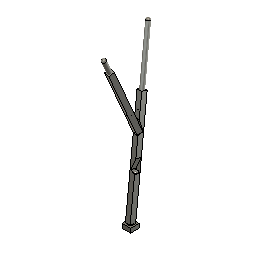
TT-4 (Autodesk Fusion 360 design; units mm, degrees)
Autodesk Fusion 360 part; units mm, degrees
sketch "Sketch1" plane through (0, 0, 0) normal (0, 1, 0) x (1, 0, 0) in component "TT-2 v5"
  line L0 (2.5, -2.5) -> (-2.5, -2.5)
  line L1 (-2.5, -2.5) -> (-2.5, 2.5)
  line L2 (-2.5, 2.5) -> (2.5, 2.5)
  line L3 (2.5, 2.5) -> (2.5, -2.5)
  constraint horizontal L0
  constraint vertical L1
  constraint horizontal L2
  constraint vertical L3
extrude "Extrude1" add sketch "Sketch1" along normal blind 2.5 makes body 1 in component "TT-2 v5"
sketch "Sketch2" plane through (0, 0, 0) normal (0, 1, 0) x (1, 0, 0) in component "TT-2 v5"
  line L0 (1.5, -1.5) -> (-1.5, -1.5)
  line L1 (-1.5, -1.5) -> (-1.5, 1.5)
  line L2 (-1.5, 1.5) -> (1.5, 1.5)
  line L3 (1.5, 1.5) -> (1.5, -1.5)
  constraint horizontal L0
  constraint vertical L1
  constraint horizontal L2
  constraint vertical L3
extrude "Extrude2" add sketch "Sketch2" along normal blind 60 separate body makes body 2 in component "TT-2 v5"
move_body "Move1" bodies 2 to x (0.939693, -0.34202, 0) y (0.34202, 0.939693, 0) z (0, 0, 1) at (-0.0905, -0.513, 0) in component "TT-2 v5"
move_body "Move2" bodies 2 to x (1, 0, 0) y (0, 1, 0) z (0, 0, 1) at (3.3727, 9.6612, 0) in component "TT-2 v5"
sphere "SpherePrimitive1" add diameter 3 placed x (0, 0, 1) y (-0.939693, 0.34202, 0) z (-0.34202, -0.939693, 0) at (3.3241, 9.1329, 0) bodies 2 in component "TT-2 v5"
sphere "SpherePrimitive2" cut diameter 3 placed x (-1, 0, 0) y (0, 0, 1) z (0, 1, 0) at (0, 2.5, 0) bodies 1 in component "TT-2 v5"
cylinder "CylinderPrimitive1" add diameter 2.5 height 40 placed x (0.883022, -0.321394, -0.34202) y (-0.321394, 0.116978, -0.939693) z (0.34202, 0.939693, 0) at (23.8453, 65.5145, 0) separate body makes body 3 in component "TT-2 v5"
sphere "SpherePrimitive3" add diameter 2.5 placed x (0, 0, -1) y (-0.939693, 0.34202, 0) z (0.34202, 0.939693, 0) at (37.5261, 103.1022, 0) bodies 3 in component "TT-2 v5"
move_body "Move3" bodies 3 2 to x (0.939693, 0.34202, 0) y (-0.34202, 0.939693, 0) z (0, 0, 1) at (23.6283, -3.8286, 0) in component "TT-2 v5"
move_body "Move4" bodies 2 3 to x (1, 0, 0) y (0, 1, 0) z (0, 0, 1) at (-23.6681, -3.196, 0) in component "TT-2 v5"
copy_body "CopyPasteBodies1" bodies 3 2 makes body 4 makes body 5 in component "TT-2 v5"
move_body "Move5" bodies 4 5 to x (1, 0, 0) y (0, 0.906308, 0.422618) z (0, -0.422618, 0.906308) at (0, 42.015, -10.6133) in component "TT-2 v5"
move_body "Move6" bodies 5 4 to x (1, 0, 0) y (0, 1, 0) z (0, 0, 1) at (0, -2.8403, 9.6134) in component "TT-2 v5"
extrude "Extrude3" cut 1 faces at (0.4157, 96.2065, 25.0427) along direction (0, -0.906308, -0.422618) blind 15 on bodies 5 bodies 5 in component "TT-2 v5"
move_body "Move7" bodies 4 to x (1, 0, 0) y (0, 1, 0) z (0, 0, 1) at (0, -26.7116, -12.4558) in component "TT-2 v5"
move_body "Move8" bodies 5 4 to x (1, 0, 0) y (0, 1, 0) z (0, 0, 1) at (0, -15.5908, 0) in component "TT-2 v5"
copy_body "CopyPasteBodies2" bodies 4 5 makes body 6 makes body 7 in component "TT-2 v5"
move_body "Move9" bodies 6 7 to x (0, 0, -1) y (0, 1, 0) z (1, 0, 0) at (-0.0791, 0, -0.06) in component "TT-2 v5"
move_body "Move10" bodies 6 to x (1, 0, 0) y (0, 1, 0) z (0, 0, 1) at (5.2397, 11.2365, 0) in component "TT-2 v5"
move_body "Move11" bodies 7 3 4 2 5 6 to x (1, 0, 0) y (0, 0.984808, -0.173648) z (0, 0.173648, 0.984808) at (0, 0.0409, 0.4679) in component "TT-2 v5"
move_body "Move12" bodies 5 4 to x (1, 0, 0) y (0, 1, 0) z (0, 0, 1) at (0, 17.3834, -3.0131) in component "TT-2 v5"
sketch "Sketch7" plane through (0, 0, 0) normal (0, 1, 0) x (1, 0, 0) in component "TT-2 v5"
  line L0 (20, -30) -> (50, 15)
  line L1 (50, 15) -> (20, 47.2574)
  line L2 (20, 47.2574) -> (-26.886, 18.4817)
  line L3 (-26.886, 18.4817) -> (-3.443, -34.2088)
  line L4 (-3.443, -34.2088) -> (20, -30)
extrude "Extrude4" add sketch "Sketch7" along normal blind 2 separate body makes body 8 in component "TT-2 v5"
move_body "Move13" bodies 8 to x (1, 0, 0) y (0, 1, 0) z (0, 0, 1) at (0, 114.7446, 0) in component "TT-2 v5"
sketch "Sketch8" plane through (0, 114.7446, 0) normal (0, -1, 0) x (1, 0, 0) in component "TT-2 v5"
  line L0 (20, 30) -> (-3.443, 34.2088)
  line L1 (-3.443, 34.2088) -> (-26.886, -18.4817)
  line L2 (-26.886, -18.4817) -> (20, -47.2574)
  line L3 (20, -47.2574) -> (50, -15)
  line L4 (50, -15) -> (20, 30)
sphere "SpherePrimitive4" cut diameter 2.5 placed x (1, 0, 0) y (0, 0, 1) z (0, -1, 0) at (-5, 114.7446, -17) bodies 8 in component "TT-2 v5"
sphere "SpherePrimitive5" cut diameter 2.5 placed x (1, 0, 0) y (0, 0, 1) z (0, -1, 0) at (3, 114.7446, 17) bodies 8 in component "TT-2 v5"
sphere "SpherePrimitive6" cut diameter 2.5 placed x (1, 0, 0) y (0, 0, 1) z (0, -1, 0) at (32.239, 114.7446, -14.3242) bodies 8 in component "TT-2 v5"
copy_body "CopyPasteBodies3" bodies 7 5 makes body 9 makes body 10 in component "TT-2 v5"
extrude "Extrude5" cut 1 faces at (19.5306, 65.7186, -10.5804) along direction (-0.422618, -0.892539, 0.157379) blind 45 on bodies 9 bodies 9 in component "TT-2 v5"
extrude "Extrude6" cut 1 faces at (-0.5843, 86.4162, 5.2019) along direction (0, -0.965926, -0.258819) blind 45 on bodies 10 bodies 10 in component "TT-2 v5"
combine "Combine1" operation cut target body 2 tool bodies 9 in component "TT-2 v5"
combine "Combine2" operation cut target body 2 tool bodies 10 in component "TT-2 v5"
copy_body "CopyPasteBodies4" bodies 7 5 makes body 11 makes body 12 in component "TT-2 v5"
combine "Combine3" operation cut target body 2 tool bodies 11 12 in component "TT-2 v5"
copy_body "Body->Comp1" bodies 1 removing the originals makes body 13 in component "MainFix"
copy_body "Body->Comp2" bodies 3 removing the originals makes body 14 in component "MainAct"
copy_body "Body->Comp3" bodies 4 removing the originals makes body 15 in component "LeftAct"
copy_body "Body->Comp4" bodies 2 removing the originals makes body 16 in component "MainBranch"
copy_body "Body->Comp5" bodies 5 removing the originals makes body 17 in component "LeftBranch"
component "TT-2 v5" placed x (1, 0, 0) y (0, 1, 0) z (0, 0, 1) at (0, 0, 0)
component "MainFix" placed x (1, 0, 0) y (0, 1, 0) z (0, 0, 1) at (0, 0, 0) in component "TT-2 v5"
component "MainAct" placed x (0.989237, 0.127632, 0.071552) y (-0.124231, 0.990986, -0.050136) z (-0.077306, 0.040708, 0.996176) at (1.2805, -8.6251, 2.0751) in component "TT-2 v5"
component "LeftAct" placed x (0.981708, -0.119953, 0.147853) y (0.093376, 0.980101, 0.175163) z (-0.165923, -0.158153, 0.973374) at (-10.451, -16.2774, -16.7957) in component "TT-2 v5"
component "MainBranch" placed x (0.989237, 0.127632, 0.071552) y (-0.124231, 0.990986, -0.050136) z (-0.077306, 0.040708, 0.996176) at (0.3741, -0.1651, 0.1379) in component "TT-2 v5"
component "LeftBranch" placed x (0.981708, -0.119953, 0.147853) y (0.093376, 0.980101, 0.175163) z (-0.165923, -0.158153, 0.973374) at (-9.6144, -1.0838, -9.7226) in component "TT-2 v5"
hidden bodies 7 6 8
named bodies: "MainFix", "MainBranch", "MainAct", "LeftAct", "LeftBranch", "MainAct (1)", "MainBranch (1)", "RightAct", "RightBranch", "Flat", "RightBranch (1)", "LeftBranch (1)"
